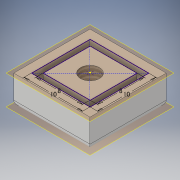
# Autodesk Inventor part: pin_joint_ver1
Saved by Autodesk Inventor 2019.3 (Build 233278000, 278)
## iProperties
Created: 2019-08-27
Part Number: pin_joint_ver1
Material: Generic
Document SubType Name: Modeling
Designer: ushiyama
Density: 1 g/cm^3
Appearance: Default
Author: ushiyama
Autodesk Inventor part; units mm, degrees
ref_plane "YZ Plane" through (0, 0, 0) normal (1, 0, 0) x (0, 1, 0)
ref_plane "XY Plane" through (0, 0, 0) normal (0, 0, 1) x (1, 0, 0)
sketch "スケッチ1" plane through (0, 0, 0) normal (0, 1, 0) x (-1, 0, 0)
  line L0 (6.5, -6.5) -> (-6.5, -6.5)
  line L1 (-6.5, -6.5) -> (-6.5, 6.5)
  line L2 (-6.5, 6.5) -> (6.5, 6.5)
  line L3 (6.5, 6.5) -> (6.5, -6.5)
  line L4 (6.5, -6.5) -> (-6.5, 6.5) construction
  line L5 (-6.5, -6.5) -> (6.5, 6.5) construction
  dimension "d1" = 13
  dimension "d2" = 13
  constraints: 12 end point, 2 parallel, 1 horizontal, 1 perpendicular
  measures "d1" distance of L1.end L2.end
  measures "d2" distance of L0.end L1.end
extrude "押し出し4" add sketch "スケッチ1" along normal blind 5
ref_plane "作業平面2" through (0, 5, 0) normal (0, 1, 0) x (-1, 0, 0)
sketch "スケッチ3" plane through (0, 5, 0) normal (0, 1, 0) x (-1, 0, 0)
  line L0 (4, -4) -> (-4, -4)
  line L1 (-4, -4) -> (-4, 4)
  line L2 (-4, 4) -> (4, 4)
  line L3 (4, 4) -> (4, -4)
  line L4 (4, -4) -> (-4, 4) construction
  line L5 (-4, -4) -> (4, 4) construction
  line L6 (5, -5) -> (-5, -5)
  line L7 (-5, -5) -> (-5, 5)
  line L8 (-5, 5) -> (5, 5)
  line L9 (5, 5) -> (5, -5)
  line L10 (5, -5) -> (-5, 5) construction
  line L11 (-5, -5) -> (5, 5) construction
  point P0 (0, 0)
  point P1 (0, 0)
  dimension "d19" = 8
  dimension "d20" = 8
  dimension "d21" = 10
  dimension "d22" = 10
  constraints: 24 end point, 4 midpoint, 4 parallel, 2 horizontal, 2 perpendicular, 1 coincident
  measures "d19" distance of L1.end L2.end
  measures "d20" distance of L0.end L1.end
  measures "d21" distance of L7.end L8.end
  measures "d22" distance of L6.end L7.end
extrude "押し出し5" cut sketch "スケッチ3" against normal blind 3
hole "穴1" at (0, 5, 0) direction (0, -1, 0) diameter 3.242 end through all thread size "M4x0.7" class "6H" standard "ANSI Metric M Profile"
fillet "フィレット1" radius 1 4 edges at (0, 0, -6.5) (6.5, 0, 0) (-6.5, 0, 0) (0, 0, 6.5)
sketch "スケッチ4" plane through (0, 5, 0) normal (0, 1, 0) x (1, 0, 0)
  point P0 (0, 0)
sketch "スケッチ5" plane through (0, 5, 0) normal (0, 1, 0) x (1, 0, 0)
  point P0 (0, 0)
